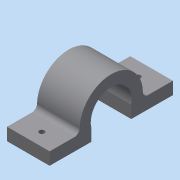
# Autodesk Inventor part: motor mounts
Saved by Autodesk Inventor 2015 (Build 190159000, 159)
## iProperties
Created: 2015-06-24
Part Number: motor mounts
Material: Generic
Document SubType Name: Modeling
Designer: Rahul
Density: 1 g/cm^3
Appearance: Default
Author: Rahul
Autodesk Inventor part; units mm, degrees
ref_plane "YZ Plane" through (0, 0, 0) normal (1, 0, 0) x (0, 1, 0)
ref_plane "XZ Plane" through (0, 0, 0) normal (0, 1, 0) x (-1, 0, 0)
ref_plane "XY Plane" through (0, 0, 0) normal (0, 0, 1) x (1, 0, 0)
sketch "Sketch1" plane through (0, 0, 0) normal (0, 0, 1) x (1, 0, 0)
  line L0 (-37.6, 3.81) -> (-12.2, 3.81)
  line L1 (-12.2, 3.81) -> (-12.2, -3.81)
  line L2 (-12.2, -3.81) -> (-37.6, -3.81)
  line L3 (-37.6, -3.81) -> (-37.6, 3.81)
  line L4 (-52.64, 0) -> (52.64, 0) projected
  line L5 (0, -32.0572) -> (0, 10.9036) projected
  line L6 (12.2, 3.81) -> (37.6, 3.81)
  line L7 (37.6, 3.81) -> (37.6, -3.81)
  line L8 (37.6, -3.81) -> (12.2, -3.81)
  line L9 (12.2, -3.81) -> (12.2, 3.81)
  line L10 (-9.3568, 0) -> (3.5049, 0)
  arc A0 (-12.2, -3.81) -> (12.2, -3.81) centre (0, -6.6323) ccw
  arc A1 (-19.08, -3.81) -> (19.08, -3.81) centre (0, -6.6323) ccw
  point P0 (0, 0)
  dimension "d0" = 7.62
  dimension "d2" = 7.62
  dimension "d19" = 25.4
  dimension "d20" = 25.4
  dimension "d31" = 24.4
  dimension "d32" = 12.5222
  constraints: 18 end point, 4 parallel, 4 point on circle, 2 centre point, 2 horizontal, 2 perpendicular, 2 point on line, 1 concentric, 4 other
  measures "d0" distance of L0.end L1.end
  measures "d2" distance of L6.end L7.end
  measures "d19" distance of L6.start L6.end
  measures "d20" distance of L0.start L0.end
  measures "d31" distance of L8.end L1.end
  measures "d32" radius of A0
extrude "Extrusion3" add sketch "Sketch1" along normal blind 26 contours L0 L1 L4 L3 | L4 L1 L2 L3 | L9 L4 L7 L8 | L9 L6 L7 L4
extrude "Extrusion6" add sketch "Sketch1" along normal blind 26 contours A0 L5 A1 L2 | A0 L8 A1 L5
sketch "Sketch5" plane through (-37.6, 3.81, 0) normal (0, 1, 0) x (1, 0, 0)
  circle A0 centre (7.9375, -12.7) radius 1.5875
  circle A1 centre (66.675, -12.7) radius 1.5875
  point P0 (37.6, 0)
  constraints: 2 centre point
extrude "Extrusion8" cut sketch "Sketch5" against normal blind 10.16
sketch "Sketch6" plane through (0, 0, 0) normal (0, 0, -1) x (-1, 0, 0)
  circle A0 centre (0.0788, -7.3494) radius 12.1158
  dimension "d33" = 24.2316
  constraints: 1 centre point
  measures "d33" diameter of A0
fillet "Fillet4" radius 3.175 2 edges at (-19.08, -3.81, 13) (19.08, -3.81, 13)
equation "\"d2\" = d0"
body "Solid2"
